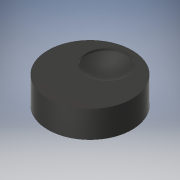
# Autodesk Inventor part: Hopper Rotary
Saved by Autodesk Inventor 2018 (Build 220112000, 112)
## iProperties
Created: 2013-10-28
Part Number: Hopper Rotary
Material: Nylon 6/6
Document SubType Name: Modeling
Designer: Gabriel Smolnycki
Mass: 4.11482 g
Surface Area: 17.3108 cm^2
Volume: 3.64143 cm^3
Density: 1.13 g/cm^3
Appearance: Smooth - Black
Sending System: SolidWorks 2017
Last Author: Gabriel Smolnycki
Last Saved: 2017-09-14
Author: Gabriel Smolnycki
Autodesk Inventor part; units mm, degrees
ref_plane "YZ Plane" through (0, 0, 0) normal (1, 0, 0) x (0, 1, 0)
ref_plane "XZ Plane" through (0, 0, 0) normal (0, 1, 0) x (-1, 0, 0)
sketch "Sketch1" plane through (0, 0, 0) normal (0, 1, 0) x (-1, 0, 0)
  circle A0 centre (0, 0) radius 12.5
  constraints: 1 centre point
extrude "Extrusion2" add sketch "Sketch1" along normal blind 8
ref_plane "Work Plane1" through (0, 0, -5) normal (0, 0, 1) x (1, 0, 0)
sketch "Sketch2" plane through (0, 0, -5) normal (0, 0, 1) x (1, 0, 0)
  arc A0 (-6, 7.5) -> (0, 5.5) centre (0, 15.5) ccw
  line L0 (-6, 8) -> (-6, 7.5)
  line L1 (-6, 8) -> (0, 8)
  line L2 (0, 5.5) -> (0, 8)
  line L3 (0, 7.5) -> (0, 17.5)
  constraints: 8 end point, 3 vertical, 2 point on circle, 1 centre point, 1 collinear, 1 horizontal
revolve "Revolution1" cut sketch "Sketch2" angle 360 about axis through (0, 7.5, -5) along (0, 1, 0)
sketch "Sketch3" plane through (0, 0, 0) normal (0, 1, 0) x (-1, 0, 0)
  line L0 (2.8583, 1.2) -> (-2.8583, 1.2)
  arc A0 (-2.8583, 1.2) -> (2.8583, 1.2) centre (0, 0) ccw
  constraints: 2 end point, 2 point on circle, 1 centre point, 1 horizontal
extrude "Extrusion1" cut sketch "Sketch3" along normal blind 5
body "Solid3"
